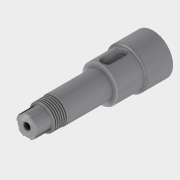
# Autodesk Inventor part: PWTR-0035
Saved by Autodesk Inventor 2021.1 (Build 251245000, 245)
## iProperties
Shininess: 64.0
Length Units: 11269
Angle Units: 11279
Time Units: 11290
Mass Units: 11284
Length Display Precision: 3
Angle Display Precision: 2
Compacted: True
Part Number: PWTR-0035
Document SubType Name: Modeling
Created: 2003-02-05
Designer: B. BOGAN
Material: Stainless Steel, 303
Description: Lower Shaft
Density: 7.75 g/cm^3
Mass: 349.76 g
Surface Area: 146.844 cm^2
Volume: 45.1303 cm^3
Appearance: Metal-Steel (Polished)
Vendor: Non-Design Specific
Density: 0.0
Volumn: 0.0
Area: 0.0
PropertySet Name: Model Information
Control State: 0
Master: False
Checked Out: False
Title: LOWER UNIVERSAL
Author: B. BOGAN
Revision Number: B
Autodesk Inventor part; units mm, degrees
ref_plane "YZ Plane" through (0, 0, 0) normal (1, 0, 0) x (0, 1, 0)
ref_plane "Offsets" through (0, 0, 50) normal (0, 0, 1) x (1, 0, 0)
ref_plane "Work Plane4" through (0, 0, 25) normal (0, 0, 1) x (1, 0, 0)
sketch "Sketch1" plane through (0, 0, 0) normal (0, 0, 1) x (1, 0, 0)
  circle A0 centre (0, 0) radius 19.0246
  dimension "d0" = 38.0492
  constraints: 1 centre point
  measures "d0" diameter of A0
extrude "Extrusion1" add sketch "Sketch1" along normal blind 100
sketch "Sketch2" plane through (0, 0, 100) normal (0, 0, 1) x (1, 0, 0)
  circle A0 centre (0, 0) radius 19.0246 projected
  circle A1 centre (0, 0) radius 17
  dimension "d3" = 34
  constraints: 1 centre point, 1 coincident, 1 concentric
  measures "d3" diameter of A1
extrude "Extrusion2" cut sketch "Sketch2" against normal up to surface (75 mm away)
sketch "Sketch8" plane through (0, 0, 100) normal (0, 0, 1) x (1, 0, 0)
  circle A0 centre (0, 0) radius 17 projected
  circle A1 centre (0, 0) radius 12.5
  dimension "d75" = 25
  constraints: 1 centre point
  measures "d75" diameter of A1
extrude "Extrusion7" cut sketch "Sketch8" against normal up to surface (50 mm away)
sketch "Sketch3" plane through (0, 0, 0) normal (0, 0, -1) x (-1, 0, 0)
  circle A0 centre (0, 0) radius 19.0246 projected
hole "Hole1" at (0, 0, 0) direction (0, 0, 1) diameter 12 depth 50 tip angle 118
sketch "Sketch4" plane through (0, 0, 0) normal (0, 1, 0) x (-1, 0, 0)
  line L0 (-19.0246, 0) -> (19.0246, 0) projected
  line L1 (3.25, 44.15) -> (3.25, 30.65)
  line L2 (-3.25, 30.65) -> (-3.25, 44.15)
  arc A0 (-3.25, 30.65) -> (3.25, 30.65) centre (0, 30.65) ccw
  arc A1 (3.25, 44.15) -> (-3.25, 44.15) centre (0, 44.15) ccw
  line L3 (0, -9.83) -> (0, 58.98) projected
  line L4 (-5, 44.15) -> (-5, 30.65)
  arc A2 (-5, 30.65) -> (5, 30.65) centre (0, 30.65) ccw
  line L5 (5, 30.65) -> (5, 44.15)
  arc A3 (5, 44.15) -> (-5, 44.15) centre (0, 44.15) ccw
  point P0 (-19.0246, 25.4)
  point P1 (19.0246, 25.4)
  dimension "d13" = 6.5
  dimension "d15" = 20
  dimension "d76" = 5
  constraints: 8 end point, 8 point on circle, 4 centre point, 4 tangent, 2 parallel, 2 point on line, 3 other
  measures "d13" distance between parallel lines of L1 L2
  measures "d76" radius of A2
extrude "Extrusion3" cut sketch "Sketch4" along normal through all both and the other way through all contours L1 A0 L3 A1 | L3 A0 L2 A1
sketch "Sketch9" plane through (0, 0, 0) normal (0, 0, -1) x (-1, 0, 0)
  circle A0 centre (0, 0) radius 19.0246 projected
  circle A1 centre (0, 0) radius 12.7 construction
  point P0 (-12.7, 0)
  dimension "d49" = 25.4
  constraints: 1 coincident, 1 horizontal alignment, 2 other
hole "Hole3" at (12.7, 0, 0) direction (0, 0, 1) diameter 3.937 depth 19.05 tip angle 118 thread size "10-24 UNC" class "2B" standard "ANSI Unified Screw Threads"
pattern_circular "Circular Pattern1" count 4 over 360 about axis through (0, 0, 25) along (0, 0, -1) of "Hole3"
ref_plane "Work Plane3" through (0, 17, 100) normal (0, 1, 0) x (-1, 0, 0)
extrude "Extrusion12" cut sketch "Sketch4" against normal blind 5 from surface at 17
sketch "Sketch12" plane through (0, 0, 100) normal (0, 0, 1) x (1, 0, 0)
  circle A0 centre (0, 0) radius 10
  circle A1 centre (0, 0) radius 9
  line L0 (-3.0902, 9.5106) -> (-3.0902, 8.4529) construction
  line L1 (3.0902, 9.5106) -> (3.0902, 8.4529) construction
  line L2 (-3.0902, 9.5106) -> (0, 0)
  line L3 (0, 0) -> (3.0902, 9.5106)
  point P0 (2.7812, 8.5595)
  point P1 (-2.7812, 8.5595)
  dimension "d85" = 20
  dimension "d98" = 18
  dimension "d112" = 36
  constraints: 8 end point, 4 point on circle, 2 centre point, 2 coincident, 2 parallel, 1 vertical
  measures "d85" diameter of A0
  measures "d98" diameter of A1
  measures "d112" angle of L3 L2
sketch "Sketch15" plane through (0, 0, 100) normal (0, 0, 1) x (1, 0, 0)
  circle A0 centre (0, 0) radius 12
  circle A1 centre (0, 0) radius 12.5 projected
  dimension "d113" = 24
  constraints: 1 centre point, 1 coincident
  measures "d113" diameter of A0
extrude "Extrusion15" cut sketch "Sketch15" against normal blind 12
thread "Thread1" size "M24x2" class "6g" standard "ISO Metric profile" full length
extrude "Extrusion13" add sketch "Sketch12" along normal blind 14.5 contours L3 L2 A1 | A1 L2 L3
extrude "Extrusion14" add sketch "Sketch12" along normal up to surface (14.5 mm away) contours L3 A1 L2 A0 picked at (1.6921, 9.4688)
pattern_circular "Circular Pattern2" count 5 over 360 about axis through (0, 0, -10) along (0, 0, 1) of "Extrusion14"
sketch "Sketch14" plane through (0, 0, 114.5) normal (0, 0, 1) x (1, 0, 0)
  point P0 (0, 0)
  point P1 (0, 0)
  point P2 (0, 0)
  constraints: 1 coincident
hole "Hole6" at (0, 0, 114.5) direction (0, 0, -1) diameter 6.647 depth 22.2 tip angle 118 thread size "M8x1.25" class "6H" standard "ISO Metric profile"
body "Solid1"
